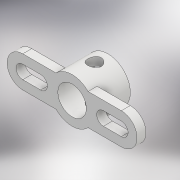
# Autodesk Inventor part: EncoderWheelAdapterSlotted
Saved by Autodesk Inventor 2018.2 (Build 222227000, 227)
## iProperties
Created: 2018-03-25
Part Number: EncoderWheelAdapterSlotted
Material: ABS Plastic
Document SubType Name: Modeling
Designer: mansu
Density: 1.06 g/cm^3
Appearance: Smooth - White
Mass: 0.492256 g
Surface Area: 7.06553 cm^2
Volume: 0.464392 cm^3
Author: mansu
Autodesk Inventor part; units mm, degrees
ref_plane "YZ Plane" through (0, 0, 0) normal (1, 0, 0) x (0, 1, 0)
ref_plane "XZ Plane" through (0, 0, 0) normal (0, 1, 0) x (-1, 0, 0)
sketch "Sketch1" plane through (0, 0, 0) normal (0, 1, 0) x (-1, 0, 0)
  circle A0 centre (0, 0) radius 3.175
  arc A1 (4.1151, 2.84) -> (3.5707, 3.5) centre (0, 0) ccw
  arc A2 (-11, 3.5) -> (-11, -3.5) centre (-11, 0) ccw
  line L0 (0, 0) -> (0, -5) construction
  arc A3 (4.1151, -2.84) -> (4.1151, 2.84) centre (0, 0) ccw
  line L1 (-7, 0) -> (-11, 0) construction
  line L2 (-7, -1.5) -> (-11, -1.5)
  line L3 (-11, 1.5) -> (-7, 1.5)
  arc A4 (-7, -1.5) -> (-7, 1.5) centre (-7, 0) ccw
  arc A5 (-11, 1.5) -> (-11, -1.5) centre (-11, 0) ccw
  line L4 (-11, 3.5) -> (-3.5707, 3.5)
  line L5 (-11, -3.5) -> (-3.5707, -3.5)
  line L6 (0, 0) -> (0, 3.175) construction
  arc A6 (11, -3.5) -> (11, 3.5) centre (11, 0) ccw
  line L7 (7, -1.5) -> (11, -1.5)
  line L8 (11, 1.5) -> (7, 1.5)
  arc A7 (7, 1.5) -> (7, -1.5) centre (7, 0) ccw
  arc A8 (11, -1.5) -> (11, 1.5) centre (11, 0) ccw
  line L9 (11, 3.5) -> (3.5707, 3.5)
  line L10 (11, -3.5) -> (3.5707, -3.5)
  arc A9 (3.5707, 3.5) -> (3.5707, -3.5) centre (0, 0) ccw
  arc A10 (3.5707, -3.5) -> (4.1151, -2.84) centre (0, 0) ccw
  point P0 (-9, 0)
  dimension "d0" = 6.35
  dimension "d1" = 10
  dimension "d6" = 3.5
  dimension "d15" = 3
  dimension "d16" = 4
  dimension "d17" = 7
  constraints: 29 point on circle, 24 end point, 10 centre point, 10 symmetric about line, 6 tangent, 3 horizontal, 2 coincident, 2 vertical, 1 horizontal alignment, 1 midpoint, 1 parallel, 1 vertical alignment, 5 other
  measures "d1" diameter of A1
  measures "d6" radius of A2
  measures "d15" distance between parallel lines of L3 L2
  measures "d16" distance of L1.start L1.end
  measures "d17" distance of point (0, 0) L1.start
extrude "Extrusion1" add sketch "Sketch1" against normal blind 2
extrude "Extrusion2" add sketch "Sketch1" along normal blind 6 contours A3 A10 A9 A1
sketch "Sketch2" plane through (0, 0, 0) normal (0, 0, 1) x (1, 0, 0)
  circle A0 centre (0, 3) radius 1.5
  line L0 (5, 6) -> (5, 0) projected
  point P0 (0, 0)
  point P1 (5, 3)
  dimension "d11" = 3
  constraints: 1 centre point, 1 horizontal alignment, 1 midpoint, 1 vertical alignment
  measures "d11" diameter of A0
extrude "Extrusion3" cut sketch "Sketch2" along normal through all both and the other way through all
ref_plane "Work Plane1" through (0, 0, 5) normal (0, 0, 1) x (1, 0, 0)
body "Solid1"
